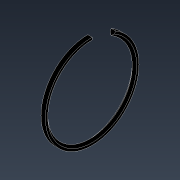
# Autodesk Inventor part: Pierścień klinowy
Saved by Autodesk Inventor 2022 (Build 260153000, 153)
## iProperties
Created: 2023-05-24
Part Number: Pierścień klinowy
Material: Generic
Document SubType Name: Modeling
Designer: wikto
Density: 1 g/cm^3
Appearance: Anodized - Black
Author: wikto
Autodesk Inventor part; units mm, degrees
ref_plane "YZ Plane" through (0, 0, 0) normal (1, 0, 0) x (0, 1, 0)
ref_plane "XZ Plane" through (0, 0, 0) normal (0, 1, 0) x (-1, 0, 0)
ref_plane "XY Plane" through (0, 0, 0) normal (0, 0, 1) x (1, 0, 0)
sketch "Sketch1" plane through (0, 0, 0) normal (0, 0, 1) x (1, 0, 0)
  line L0 (0, 27.0856) -> (-1.414, 28.5)
  line L1 (-1.414, 28.5) -> (-1.414, 30)
  line L2 (-1.414, 30) -> (1.414, 30)
  line L3 (1.414, 30) -> (1.414, 28.5)
  line L4 (1.414, 28.5) -> (0, 27.0856)
  line L5 (-5, 0) -> (5, 0)
  point P0 (0, 0)
  point P1 (0, 30)
  point P2 (0, 0)
  dimension "d0" = 2
  dimension "d1" = 10
  dimension "d3" = 57
  dimension "d4" = 2.828
  dimension "d5" = 1.5
  constraints: 12 end point, 2 equal length, 2 midpoint, 2 perpendicular, 1 coincident, 1 horizontal, 1 vertical, 1 vertical alignment
  measures "d0" distance of L3.end L0.start
  measures "d1" distance of L5.start L5.end
  measures "d3" diameter of L3.end L5
  measures "d4" distance between parallel lines of L1 L3
  measures "d5" distance of L2.end L3.end
revolve "Revolution1" add sketch "Sketch1" angle 330 about axis through (-5, 0, 0) along (1, 0, 0)
body "Solid1"
